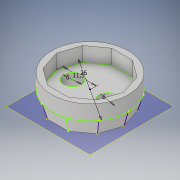
# Autodesk Inventor part: Probe P1.5
Saved by Autodesk Inventor 2019 (Build 230136000, 136)
## iProperties
Created: 2019-07-29
Part Number: Probe P1.5
Material: Generic
Document SubType Name: Modeling
Designer: azriel
Density: 1 g/cm^3
Appearance: Default
Author: azriel
Autodesk Inventor part; units mm, degrees
ref_plane "YZ Plane" through (0, 0, 0) normal (1, 0, 0) x (0, 1, 0)
ref_plane "XZ Plane" through (0, 0, 0) normal (0, 1, 0) x (-1, 0, 0)
ref_plane "XY Plane" through (0, 0, 0) normal (0, 0, 1) x (1, 0, 0)
sketch "Sketch1" plane through (0, 0, 0) normal (0, 1, 0) x (-1, 0, 0)
  circle A0 centre (0, 0) radius 13
  line L0 (-11.5, 0) -> (-9.303695, 6.75953) construction
  line L1 (-9.303695, 6.75953) -> (-3.553695, 10.93715) construction
  line L2 (-3.553695, 10.93715) -> (3.553695, 10.93715) construction
  line L3 (3.553695, 10.93715) -> (9.303695, 6.75953) construction
  line L4 (9.303695, 6.75953) -> (11.5, 0) construction
  line L5 (11.5, 0) -> (9.303695, -6.75953) construction
  line L6 (9.303695, -6.75953) -> (3.553695, -10.93715) construction
  line L7 (3.553695, -10.93715) -> (-3.553695, -10.93715) construction
  line L8 (-3.553695, -10.93715) -> (-9.303695, -6.75953) construction
  line L9 (-9.303695, -6.75953) -> (-11.5, 0) construction
  circle A1 centre (-6, 0) radius 3 construction
  circle A2 centre (6, 0) radius 3 construction
  line L10 (13, 0) -> (10.517221, -7.641208) construction
  line L11 (10.517221, -7.641208) -> (4.017221, -12.363735) construction
  line L12 (4.017221, -12.363735) -> (-4.017221, -12.363735) construction
  line L13 (-4.017221, -12.363735) -> (-10.517221, -7.641208) construction
  line L14 (-10.517221, -7.641208) -> (-13, 0) construction
  line L15 (-13, 0) -> (-10.517221, 7.641208) construction
  line L16 (-10.517221, 7.641208) -> (-4.017221, 12.363735) construction
  line L17 (-4.017221, 12.363735) -> (4.017221, 12.363735) construction
  line L18 (4.017221, 12.363735) -> (10.517221, 7.641208) construction
  line L19 (10.517221, 7.641208) -> (13, 0) construction
  dimension "d0" = 26
  dimension "d10" = 6
  dimension "d11" = 6
  constraints: 40 end point, 2 centre point, 2 coincident, 1 horizontal alignment, 23 other
  measures "d10" diameter of A1
  measures "d11" diameter of A2
ref_plane "Work Plane1" through (0, -5, 0) normal (0, -1, 0) x (1, 0, 0)
sketch "Sketch2" plane through (0, -5, 0) normal (0, -1, 0) x (1, 0, 0)
  circle A0 centre (0, 0) radius 13 construction
  line L0 (-9.303695, 6.75953) -> (-11.5, 0)
  line L1 (-11.5, 0) -> (-9.303695, 6.75953)
  line L2 (-9.303695, 6.75953) -> (-3.553695, 10.93715)
  line L3 (-3.553695, 10.93715) -> (3.553695, 10.93715)
  line L4 (3.553695, 10.93715) -> (9.303695, 6.75953)
  line L5 (9.303695, 6.75953) -> (11.5, 0)
  line L6 (11.5, 0) -> (9.303695, -6.75953)
  line L7 (9.303695, -6.75953) -> (3.553695, -10.93715)
  line L8 (3.553695, -10.93715) -> (-3.553695, -10.93715)
  line L9 (-3.553695, -10.93715) -> (-9.303695, -6.75953)
  line L10 (-9.303695, -6.75953) -> (-11.5, 0)
  constraints: 20 end point, 2 coincident, 1 centre point, 21 other
sketch3d "3D Sketch1"
sketch "Sketch1 outline for Loft1" plane through (0, 0, 0) normal (0, 1, 0) x (-1, 0, 0)
  circle A0 centre (0, 0) radius 13
sketch "Sketch2 outline for Loft1" plane through (0, -5, 0) normal (0, -1, 0) x (1, 0, 0)
  line L0 (-11.5, 0) -> (-9.303695, 6.75953)
  line L1 (-9.303695, 6.75953) -> (-3.553695, 10.93715)
  line L2 (-3.553695, 10.93715) -> (3.553695, 10.93715)
  line L3 (3.553695, 10.93715) -> (9.303695, 6.75953)
  line L4 (9.303695, 6.75953) -> (11.5, 0)
  line L5 (11.5, 0) -> (9.303695, -6.75953)
  line L6 (9.303695, -6.75953) -> (3.553695, -10.93715)
  line L7 (3.553695, -10.93715) -> (-3.553695, -10.93715)
  line L8 (-3.553695, -10.93715) -> (-9.303695, -6.75953)
  line L9 (-9.303695, -6.75953) -> (-11.5, 0)
loft "Loft1" add profiles "Sketch1 outline for Loft1", "Sketch2 outline for Loft1"
sketch "Sketch3" plane through (0, 0, 0) normal (0, 1, 0) x (1, 0, 0)
  circle A0 centre (0, 0) radius 13
  line L0 (-11.5, 0) -> (-9.303695, 6.75953)
  line L1 (-9.303695, 6.75953) -> (-3.553695, 10.93715)
  line L2 (-3.553695, 10.93715) -> (3.553695, 10.93715)
  line L3 (3.553695, 10.93715) -> (9.303695, 6.75953)
  line L4 (9.303695, 6.75953) -> (11.5, 0)
  line L5 (11.5, 0) -> (9.303695, -6.75953)
  line L6 (9.303695, -6.75953) -> (3.553695, -10.93715)
  line L7 (3.553695, -10.93715) -> (-3.553695, -10.93715)
  line L8 (-3.553695, -10.93715) -> (-9.303695, -6.75953)
  line L9 (-9.303695, -6.75953) -> (-11.5, 0)
  circle A1 centre (0, 0) radius 13
  line L10 (-11.5, 0) -> (-9.303695, 6.75953)
  line L11 (-9.303695, 6.75953) -> (-3.553695, 10.93715)
  line L12 (-3.553695, 10.93715) -> (3.553695, 10.93715)
  line L13 (3.553695, 10.93715) -> (9.303695, 6.75953)
  line L14 (9.303695, 6.75953) -> (11.5, 0)
  line L15 (11.5, 0) -> (9.303695, -6.75953)
  line L16 (9.303695, -6.75953) -> (3.553695, -10.93715)
  line L17 (3.553695, -10.93715) -> (-3.553695, -10.93715)
  line L18 (-3.553695, -10.93715) -> (-9.303695, -6.75953)
  line L19 (-9.303695, -6.75953) -> (-11.5, 0)
  circle A2 centre (-6, 0) radius 3
  circle A3 centre (6, 0) radius 3
  dimension "d28" = 11.5
  dimension "d29" = 26
  dimension "d30" = 6
  dimension "d31" = 6
  constraints: 40 end point, 4 centre point, 3 coincident, 21 other
  measures "d28" distance of L0.start point (0, 0)
  measures "d29" diameter of A1
  measures "d30" diameter of A2
  measures "d31" diameter of A3
extrude "Extrusion4" cut sketch "Sketch3" against normal blind 5 contours A3
extrude "Extrusion5" cut sketch "Sketch3" against normal blind 5 contours A2
extrude "Extrusion6" add sketch "Sketch3" along normal blind 5 contours A0
body "Solid2"
